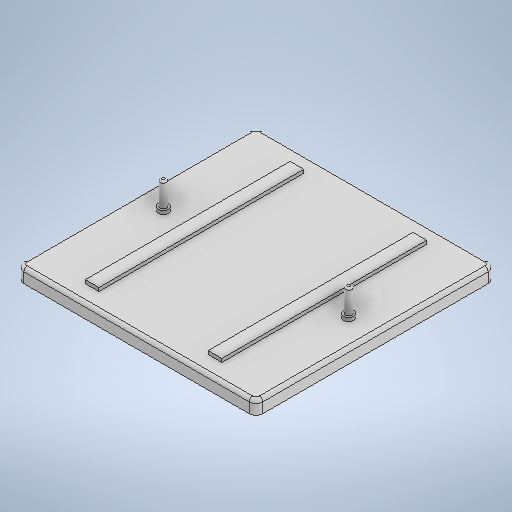
# Autodesk Inventor part: Installation Base
Saved by Autodesk Inventor 2025 (Build 290162000, 162)
## iProperties
Created: 2025-02-28
Part Number: Installation Base
Material: Generic
Document SubType Name: Modeling
Designer: Caleb Fangmeier
Density: 1 g/cm^3
Appearance: Default
Author: Caleb Fangmeier
Autodesk Inventor part; units mm, degrees
ref_plane "YZ Plane" through (0, 0, 0) normal (1, 0, 0) x (0, 1, 0)
ref_plane "XZ Plane" through (0, 0, 0) normal (0, 1, 0) x (-1, 0, 0)
ref_plane "XY Plane" through (0, 0, 0) normal (0, 0, 1) x (1, 0, 0)
sketch "Sketch1" plane through (0, 0, 0) normal (0, 1, 0) x (-1, 0, 0)
  line L0 (-35, -35) -> (35, -35)
  line L1 (35, -35) -> (35, 35)
  line L2 (35, 35) -> (-35, 35)
  line L3 (-35, 35) -> (-35, -35)
  line L4 (-35, -35) -> (35, 35) construction
  line L5 (35, -35) -> (-35, 35) construction
  point P0 (0, 0)
  dimension "d0" = 70
  dimension "d1" = 70
  constraints: 12 end point, 2 midpoint, 2 parallel, 1 horizontal, 1 perpendicular
  measures "d0" distance of L0.end L1.end
  measures "d1" distance of L1.end L2.end
extrude "Extrusion1" add sketch "Sketch1" along normal blind 4
sketch "Sketch2" plane through (0, 4, 0) normal (0, 1, 0) x (1, 0, 0)
  circle A0 centre (-27.15, 0) radius 0.9
  circle A1 centre (27.15, 0) radius 0.9
  point P0 (0, 0)
  dimension "d4" = 1.8
  dimension "d5" = 1.8
  dimension "d6" = 54.3
  dimension "d7" = 27.15
  constraints: 2 centre point, 2 horizontal alignment
  measures "d4" diameter of A0
  measures "d5" diameter of A1
  measures "d6" distance of A1.centre A0.centre
  measures "d7" distance of A0.centre point (0, 0)
extrude "Extrusion2" add sketch "Sketch2" along normal blind 8
fillet "Fillet1" radius 2 4 edges at (35, 2, 35) (-35, 2, 35) (-35, 2, -35) (35, 2, -35)
fillet "Fillet2" radius 0.5 2 edges at (26.25, 12, 0) (-28.05, 12, 0)
sketch "Sketch3" plane through (0, 4, 0) normal (0, 1, 0) x (1, 0, 0)
  circle A0 centre (27.15, 0) radius 0.9 projected
  circle A1 centre (27.15, 0) radius 1.5
  circle A2 centre (-27.15, 0) radius 0.9 projected
  circle A3 centre (-27.15, 0) radius 1.5
  line L0 (-16, -30) -> (-20, -30)
  line L1 (-20, -30) -> (-20, 30)
  line L2 (-20, 30) -> (-16, 30)
  line L3 (-16, 30) -> (-16, -30)
  line L4 (-16, -30) -> (-20, 30) construction
  line L5 (-20, -30) -> (-16, 30) construction
  line L6 (20, -30) -> (16, -30)
  line L7 (16, -30) -> (16, 30)
  line L8 (16, 30) -> (20, 30)
  line L9 (20, 30) -> (20, -30)
  line L10 (20, -30) -> (16, 30) construction
  line L11 (16, -30) -> (20, 30) construction
  point P0 (0, 0)
  point P1 (-18, 0)
  point P2 (18, 0)
  dimension "d12" = 18
  dimension "d13" = 60
  dimension "d14" = 60
  dimension "d15" = 18
  dimension "d16" = 4
  dimension "d17" = 4
  dimension "d18" = 3
  dimension "d19" = 3
  constraints: 24 end point, 4 horizontal alignment, 4 midpoint, 4 parallel, 2 centre point, 2 coincident, 2 horizontal, 2 perpendicular
  measures "d12" distance of point (0, 0) point (18, 0)
  measures "d13" distance between parallel lines of L6 L8
  measures "d14" distance of L2.end L0.start
  measures "d15" distance of point (0, 0) point (-18, 0)
  measures "d16" distance of L6.start L6.end
  measures "d17" distance of L0.start L0.end
  measures "d18" diameter of A1
  measures "d19" diameter of A3
extrude "Extrusion3" add sketch "Sketch3" along normal blind 1 contours A0 | A1 | A2 | A3 | L0 L1 L2 L3 | L6 L7 L8 L9
fillet "Fillet3" radius 1 8 edges at (34.4142, 4, 34.4142) (35, 4, 0) (34.4142, 4, -34.4142) (0, 4, -35) (-34.4142, 4, -34.4142) (-35, 4, 0) (-34.4142, 4, 34.4142) (0, 4, 35)
equation "\"d5\" = d4"
equation "\"d7\" = 0.5 * d6"
equation "\"d14\" = d13"
equation "\"d15\" = d12"
equation "\"d17\" = d16"
equation "\"d19\" = d18"
body "Solid1"
